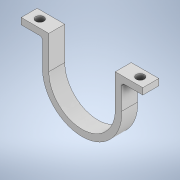
# Autodesk Inventor part: motor_support
Saved by Autodesk Inventor 2020.3 (Build 243373000, 373)
## iProperties
Created: 2020-06-21
Part Number: motor_support
Material: Generic
Document SubType Name: Modeling
Designer: Devin
Density: 1 g/cm^3
Appearance: Default
Author: Devin
Autodesk Inventor part; units mm, degrees
ref_plane "YZ Plane" through (0, 0, 0) normal (1, 0, 0) x (0, 1, 0)
ref_plane "XZ Plane" through (0, 0, 0) normal (0, 1, 0) x (-1, 0, 0)
ref_plane "XY Plane" through (0, 0, 0) normal (0, 0, 1) x (1, 0, 0)
sketch "Sketch1" plane through (0, 0, 0) normal (0, 0, 1) x (1, 0, 0)
  arc A0 (-12.5, 0) -> (12.5, 0) centre (0, 0) ccw
  line L0 (-12.5, 0) -> (-12.5, 12.5)
  line L1 (12.5, 0) -> (12.5, 12.5)
  arc A1 (-14.879, 0.7912) -> (14.879, 0.7912) centre (0, 0) ccw
  line L2 (-14.879, 0.7912) -> (-14.879, 10.1)
  line L3 (14.879, 0.7912) -> (14.879, 10.1)
  line L4 (-22.879, 12.5) -> (-22.879, 10.1)
  line L5 (-22.879, 10.1) -> (-14.879, 10.1)
  line L6 (-22.879, 12.5) -> (-12.5, 12.5)
  line L7 (22.879, 12.5) -> (22.879, 10.1)
  line L8 (22.879, 10.1) -> (14.879, 10.1)
  line L9 (22.879, 12.5) -> (12.5, 12.5)
  constraints: 20 end point, 4 perpendicular, 4 point on circle, 3 vertical, 2 centre point, 2 coincident, 2 tangent, 1 horizontal
extrude "Extrusion1" add sketch "Sketch1" along normal blind 6
sketch "Sketch2" plane through (12.5, 12.5, 0) normal (0, 1, 0) x (1, 0, 0)
  line L0 (-35.379, 0) -> (-35.379, -6) projected
  circle A0 centre (-31.379, -3) radius 1.55
  circle A1 centre (6.379, -3) radius 1.55
  line L1 (10.379, 0) -> (10.379, -6) projected
  point P0 (-12.5, 0)
  dimension "d16" = 3.1
  constraints: 2 centre point
  measures "d16" diameter of A0
extrude "Extrusion2" cut sketch "Sketch2" against normal blind 10
fillet "Fillet1" radius 1 1 edges at (14.879, 10.1, 3)
fillet "Fillet2" radius 1 1 edges at (-14.879, 10.1, 3)
body "Solid1"
